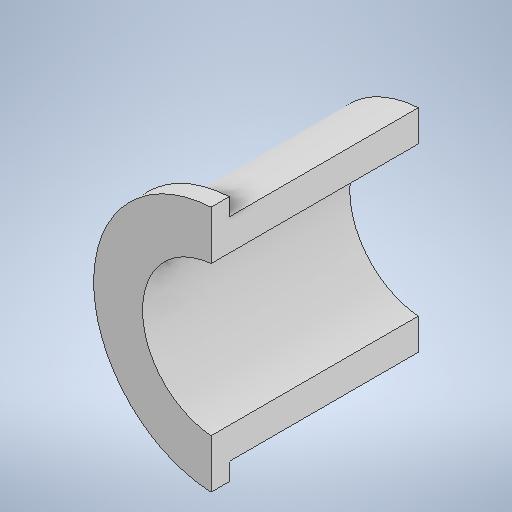
# Autodesk Inventor part: Shim
Saved by Autodesk Inventor 2025 (Build 290162000, 162)
## iProperties
Created: 2026-01-07
Part Number: Shim
Material: Generic
Document SubType Name: Modeling
Designer: tapen
Density: 1 g/cm^3
Appearance: Default
Author: tapen
Autodesk Inventor part; units mm, degrees
ref_plane "YZ Plane" through (0, 0, 0) normal (1, 0, 0) x (0, 1, 0)
ref_plane "XZ Plane" through (0, 0, 0) normal (0, 1, 0) x (-1, 0, 0)
ref_plane "XY Plane" through (0, 0, 0) normal (0, 0, 1) x (1, 0, 0)
sketch "Sketch1" plane through (0, 0, 0) normal (0, 0, 1) x (1, 0, 0)
  circle A0 centre (0, 0) radius 10.685 construction
  line L0 (-0.9, 10.647) -> (-0.9, -10.647) construction
  line L1 (-0.9, 10.647) -> (20.3941, 10.647) construction
  arc A1 (-0.9, 15.1232) -> (-0.9, -15.1232) centre (0, 0) ccw
  line L2 (-0.9, 10.647) -> (-0.9, 15.1232)
  line L3 (-0.9, -15.1232) -> (-0.9, -10.647)
  arc A2 (-0.9, 10.647) -> (-0.9, -10.647) centre (0, 0) ccw
  dimension "d0" = 21.37
  dimension "d1" = 90
  dimension "d2" = 0.9
  dimension "d3" = 15.15
  constraints: 8 end point, 6 point on circle, 3 centre point, 3 coincident, 2 perpendicular, 1 collinear, 1 horizontal
  measures "d0" diameter of A0
  measures "d1" angle of L0 L1
  measures "d2" distance from line of L0 point (0, 0)
  measures "d3" radius of A1
extrude "Extrusion1" add sketch "Sketch1" along normal blind 27
sketch "Sketch2" plane through (0, 0, 27) normal (0, 0, 1) x (1, 0, 0)
  arc A0 (-0.9, 17.627) -> (-0.9, -17.627) centre (0, 0) ccw
  arc A1 (-0.9, 15.1232) -> (-0.9, -15.1232) centre (0, 0) ccw projected
  line L0 (-0.9, 10.647) -> (-0.9, 15.1232) projected
  line L1 (-0.9, 10.647) -> (-0.9, 17.627)
  line L2 (-0.9, -17.627) -> (-0.9, -10.647)
  arc A2 (-0.9, 10.647) -> (-0.9, -10.647) centre (0, 0) ccw projected
  arc A3 (-0.9, 10.647) -> (-0.9, -10.647) centre (0, 0) ccw
  point P0 (-0.9, 15.1232)
  dimension "d6" = 17.65
  constraints: 5 point on circle, 4 end point, 2 centre point, 2 coincident, 1 collinear
  measures "d6" radius of A0
extrude "Extrusion2" add sketch "Sketch2" along normal blind 2.6
body "Solid1"
